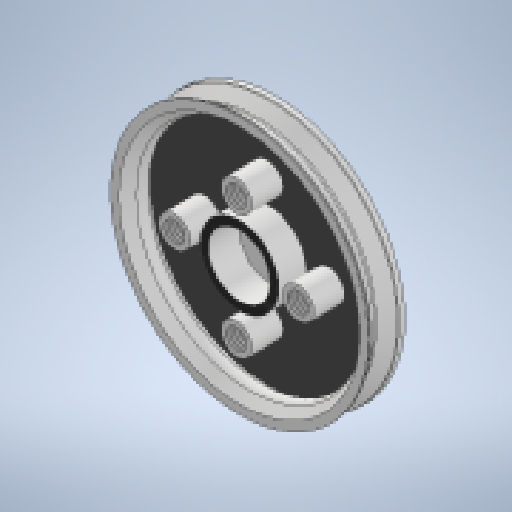
# Autodesk Inventor part: для резинки
Saved by Autodesk Inventor 2024.2 (Build 282272000, 272)
## iProperties
Created: 2025-11-25
Part Number: для резинки
Material: Типовые
Document SubType Name: Modeling
Designer: Zakhar
Density: 1 g/cm^3
Appearance: По умолчанию
Author: Zakhar
Autodesk Inventor part; units mm, degrees
ref_plane "YZ Plane" through (0, 0, 0) normal (1, 0, 0) x (0, 1, 0)
ref_plane "XZ Plane" through (0, 0, 0) normal (0, 1, 0) x (-1, 0, 0)
ref_plane "XY Plane" through (0, 0, 0) normal (0, 0, 1) x (1, 0, 0)
sketch "Эскиз1" plane through (0, 0, 0) normal (0, 1, 0) x (-1, 0, 0)
  line L0 (-12.2727, -0.6482) -> (-2.7727, -0.6482)
  line L1 (-2.7727, -0.6482) -> (-2.7727, 2.4518)
  line L2 (-2.7727, 2.4518) -> (-12.2727, 2.4518)
  line L3 (-12.2727, 2.4518) -> (-12.2727, 2.316)
  line L4 (-12.2353, 2.1996) -> (-11.3898, 1.0182)
  line L5 (-11.3898, 0.7854) -> (-12.2353, -0.396)
  line L6 (-12.2727, -0.5124) -> (-12.2727, -0.6482)
  arc A0 (-12.2727, 2.316) -> (-12.2353, 2.1996) centre (-12.0727, 2.316) ccw
  arc A1 (-12.2353, -0.396) -> (-12.2727, -0.5124) centre (-12.0727, -0.5124) ccw
  arc A2 (-11.3898, 0.7854) -> (-11.3898, 1.0182) centre (-11.5524, 0.9018) ccw
  line L7 (0.2273, 0.8513) -> (0.2273, 2.4524)
  line L8 (-2.7727, -0.6482) -> (-12.2727, -0.6482)
  line L9 (-12.2727, -0.6482) -> (-12.2727, -1.0482)
  line L10 (-12.2727, -1.0482) -> (-2.7727, -1.0482)
  line L11 (-2.7727, -1.0482) -> (-2.7727, -0.6482)
  point P0 (-12.2727, 2.2518)
  point P1 (-11.3065, 0.9018)
  point P2 (-12.2727, -0.4482)
  point P3 (-12.2727, -0.5803)
  dimension "d1" = 3.1
  dimension "d3" = 0.2
  dimension "d4" = 0.2
  dimension "d5" = 1.55
  dimension "d6" = 0.2
  dimension "d7" = 0.2
  dimension "d8" = 0.2
  dimension "d9" = 9.5
  dimension "d11" = 3
  dimension "d14" = 0.4
  constraints: 24 end point, 7 point on line, 6 point on circle, 6 tangent, 3 centre point, 3 parallel, 3 perpendicular, 2 horizontal, 2 vertical, 1 midpoint
  measures "d1" distance between parallel lines of L0 L2
  measures "d3" distance of L2.end point (-12.273, 2.252)
  measures "d4" distance of point (-12.273, -0.448) L0.start
  measures "d5" distance from line of L0 point (-11.306, 0.902)
  measures "d6" radius of A0
  measures "d7" radius of A1
  measures "d8" radius of A2
  measures "d9" distance of L1.end L2.end
  measures "d11" distance between parallel lines of L7 L1
  measures "d14" distance between parallel lines of L8 L10
revolve "Вращение2" add sketch "Эскиз1" angle 360 about axis through (-0.2273, 0, 0.8513) along (0, 0, 1)
shell "Оболочка1" thickness 0.8 removed faces 1 at (8.9849, -0.9971, 2.4518)
sketch "Эскиз2" plane through (-0.2273, 0, -1.0482) normal (0, 0, -1) x (-1, 0, 0)
  circle A0 centre (0, 0) radius 3
  point P0 (-0.2273, 0)
  dimension "d15" = 6
  constraints: 1 centre point
  measures "d15" diameter of A0
extrude "Выдавливание1" add sketch "Эскиз2" against normal blind 0.5
sketch "Эскиз3" plane through (-0.2273, 0, -0.2482) normal (0, 0, 1) x (1, 0, 0)
  circle A0 centre (-6, 0) radius 1
  circle A1 centre (-6, 0) radius 1.5
  circle A2 centre (0, 0) radius 3 projected
  line L0 (0, -3) -> (0, 2.6891) construction
  circle A3 centre (6, 0) radius 1
  circle A4 centre (6, 0) radius 1.5
  circle A5 centre (0, 6) radius 1
  circle A6 centre (0, 6) radius 1.5
  circle A7 centre (0, -6) radius 1.5
  circle A8 centre (0, -6) radius 1
  circle A9 centre (-6, 0) radius 1
  circle A10 centre (-6, 0) radius 1.5
  circle A11 centre (6, 0) radius 1.5
  circle A12 centre (6, 0) radius 1
  circle A13 centre (0, -6) radius 1
  circle A14 centre (0, -6) radius 1.5
  circle A15 centre (0, 6) radius 1.5
  circle A16 centre (0, 6) radius 1
  point P0 (0.2273, 0)
  point P1 (0, 0)
  dimension "d18" = 2
  dimension "d19" = 3
  dimension "d20" = 6
  dimension "d23" = 360
  constraints: 16 centre point, 9 coincident, 2 end point, 2 symmetric about line, 1 vertical, 1 vertical alignment, 36 other
  measures "d18" diameter of A0
  measures "d19" diameter of A1
  measures "d20" distance of point (0, 0) A0.centre
extrude "Выдавливание2" add sketch "Эскиз3" along normal blind 3 and the other way blind 4 contours A0 | A3 | A5 | A8
extrude "Выдавливание3" add sketch "Эскиз3" along normal blind 3 contours A1 | A4 | A6 | A7
equation "\"d5\" = 0.5 * d1"
